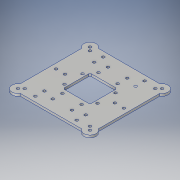
# Autodesk Inventor part: Piston Build frame
Saved by Autodesk Inventor 2018.1 (Build 221171000, 171)
## iProperties
Created: 2013-10-18
Part Number: Piston Build frame
Material: Aluminum 6061
Document SubType Name: Modeling
Designer: Gabriel Smolnycki
Mass: 160.206 g
Surface Area: 344.079 cm^2
Volume: 59.3356 cm^3
Density: 2.7 g/cm^3
Appearance: Aluminum - Flat
Sending System: SolidWorks 2017
Last Author: Gabriel Smolnycki
Last Saved: 2017-09-14
Author: Gabriel Smolnycki
Autodesk Inventor part; units mm, degrees
ref_plane "YZ Plane" through (0, 0, 0) normal (1, 0, 0) x (0, 1, 0)
ref_plane "XY Plane" through (0, 0, 0) normal (0, 0, 1) x (1, 0, 0)
ref_plane "Work Plane1" through (0, -4, 0) normal (0, 1, 0) x (-1, 0, 0)
sketch "Sketch1" plane through (0, -4, 0) normal (0, 1, 0) x (-1, 0, 0)
  arc A0 (65, 51.3397) -> (51.3397, 65) centre (60, 60) ccw
  line L0 (65, 51.3397) -> (65, -51.3397)
  arc A1 (51.3397, -65) -> (65, -51.3397) centre (60, -60) ccw
  line L1 (51.3397, -65) -> (-51.3397, -65)
  arc A2 (-65, -51.3397) -> (-51.3397, -65) centre (-60, -60) ccw
  line L2 (22.5, -20.5) -> (20.5, -22.5)
  line L3 (-65, -51.3397) -> (-65, 51.3397)
  arc A3 (-51.3397, 65) -> (-65, 51.3397) centre (-60, 60) ccw
  line L4 (22.5, 20.5) -> (22.5, -20.5)
  line L5 (20.5, 22.5) -> (22.5, 20.5)
  line L6 (-20.5, 22.5) -> (20.5, 22.5)
  line L7 (-22.5, 20.5) -> (-20.5, 22.5)
  line L8 (-51.3397, 65) -> (51.3397, 65)
  line L9 (-22.5, -20.5) -> (-22.5, 20.5)
  line L10 (-20.5, -22.5) -> (-22.5, -20.5)
  line L11 (20.5, -22.5) -> (-20.5, -22.5)
  constraints: 24 end point, 9 equal length, 8 point on circle, 4 centre point, 4 horizontal, 4 vertical, 3 equal radius, 1 perpendicular
extrude "Extrusion1" add sketch "Sketch1" along normal blind 4.064
hole "Hole32" at (34.5, 0.064, 56.5) direction (0, -1, 0) diameter 4.5 depth 4.064 tip angle 118
hole "Hole31" at (34.5, 0.064, 41.5) direction (0, -1, 0) diameter 4.5 depth 4.064 tip angle 118
hole "Hole30" at (56.5, 0.064, 0) direction (0, -1, 0) diameter 4.5 depth 4.064 tip angle 118
hole "Hole29" at (41.5, 0.064, 0) direction (0, -1, 0) diameter 4.5 depth 4.064 tip angle 118
hole "Hole28" at (34.5, 0, -41.5) direction (0, -1, 0) diameter 4.5 depth 4 tip angle 118
hole "Hole27" at (34.5, 0.064, -56.5) direction (0, -1, 0) diameter 4.5 depth 4.064 tip angle 118
hole "Hole26" at (-34.5, 0.064, -56.5) direction (0, -1, 0) diameter 4.5 depth 4.064 tip angle 118
hole "Hole25" at (-34.5, 0.064, -41.5) direction (0, -1, 0) diameter 4.5 depth 4.064 tip angle 118
hole "Hole24" at (-41.5, 0.064, 0) direction (0, -1, 0) diameter 4.5 depth 4.064 tip angle 118
hole "Hole23" at (-56.5, 0.064, 0) direction (0, -1, 0) diameter 4.5 depth 4.064 tip angle 118
hole "Hole22" at (-34.5, 0.064, 41.5) direction (0, -1, 0) diameter 4.5 depth 4.064 tip angle 118
hole "Hole21" at (-34.5, 0.064, 56.5) direction (0, -1, 0) diameter 4.5 depth 4.064 tip angle 118
hole "Hole20" at (-16, 0.064, -46) direction (0, -1, 0) diameter 4.5 depth 4.064 tip angle 118
hole "Hole19" at (-16, 0.064, -30) direction (0, -1, 0) diameter 4.5 depth 4.064 tip angle 118
hole "Hole18" at (16, 0.064, -30) direction (0, -1, 0) diameter 4.5 depth 4.064 tip angle 118
hole "Hole17" at (16, 0.064, -46) direction (0, -1, 0) diameter 4.5 depth 4.064 tip angle 118
sketch "Sketch17" plane through (0, 0.064, 0) normal (0, 1, 0) x (-1, 0, 0)
  point P0 (-16, -46)
hole "Hole16" at (16, 0.064, 46) direction (0, -1, 0) diameter 4.5 depth 4.064 tip angle 118
sketch "Sketch16" plane through (0, 0.064, 0) normal (0, 1, 0) x (-1, 0, 0)
  point P0 (-16, -30)
hole "Hole15" at (16, 0.064, 30) direction (0, -1, 0) diameter 4.5 depth 4.064 tip angle 118
sketch "Sketch15" plane through (0, 0.064, 0) normal (0, 1, 0) x (-1, 0, 0)
  point P0 (16, -30)
hole "Hole14" at (-16, 0.064, 30) direction (0, -1, 0) diameter 4.5 depth 4.064 tip angle 118
sketch "Sketch14" plane through (0, 0.064, 0) normal (0, 1, 0) x (-1, 0, 0)
  point P0 (16, -46)
hole "Hole13" at (-16, 0.064, 46) direction (0, -1, 0) diameter 4.5 depth 4.064 tip angle 118
sketch "Sketch13" plane through (0, 0.064, 0) normal (0, 1, 0) x (-1, 0, 0)
  point P0 (34.5, 56.5)
hole "Hole12" at (-27.5, 0.064, 15) direction (0, -1, 0) diameter 4.5 depth 4.064 tip angle 118
sketch "Sketch12" plane through (0, 0.064, 0) normal (0, 1, 0) x (-1, 0, 0)
  point P0 (34.5, 41.5)
hole "Hole11" at (-27.5, 0.064, -15) direction (0, -1, 0) diameter 4.5 depth 4.064 tip angle 118
sketch "Sketch11" plane through (0, 0.064, 0) normal (0, 1, 0) x (-1, 0, 0)
  point P0 (56.5, 0)
hole "Hole10" at (27.5, 0.064, -15) direction (0, -1, 0) diameter 4.5 depth 4.064 tip angle 118
sketch "Sketch10" plane through (0, 0.064, 0) normal (0, 1, 0) x (-1, 0, 0)
  point P0 (41.5, 0)
hole "Hole9" at (27.5, 0.064, 15) direction (0, -1, 0) diameter 4.5 depth 4.064 tip angle 118
sketch "Sketch9" plane through (0, 0.064, 0) normal (0, 1, 0) x (-1, 0, 0)
  point P0 (34.5, -41.5)
hole "Hole8" at (54.3431, 0.064, -54.3431) direction (0, -1, 0) diameter 4.5 depth 4.064 tip angle 118
sketch "Sketch8" plane through (0, 0.064, 0) normal (0, 1, 0) x (-1, 0, 0)
  point P0 (34.5, -56.5)
hole "Hole7" at (54.3431, 0.064, 54.3431) direction (0, -1, 0) diameter 4.5 depth 4.064 tip angle 118
sketch "Sketch7" plane through (0, 0.064, 0) normal (0, 1, 0) x (-1, 0, 0)
  point P0 (-34.5, -56.5)
hole "Hole6" at (-54.3431, 0.064, 54.3431) direction (0, -1, 0) diameter 4.5 depth 4.064 tip angle 118
sketch "Sketch6" plane through (0, 0, 0) normal (0, 1, 0) x (-1, 0, 0)
  point P0 (-34.5, -41.5)
hole "Hole5" at (-60, -4, 60) direction (0, 1, 0) diameter 4.5 depth 4.064 tip angle 118
sketch "Sketch5" plane through (0, 0.064, 0) normal (0, 1, 0) x (-1, 0, 0)
  point P0 (-41.5, 0)
hole "Hole4" at (60, -4, 60) direction (0, 1, 0) diameter 4.5 depth 4.064 tip angle 118
sketch "Sketch4" plane through (0, 0.064, 0) normal (0, 1, 0) x (-1, 0, 0)
  point P0 (-56.5, 0)
hole "Hole3" at (60, -4, -60) direction (0, 1, 0) diameter 4.5 depth 4.064 tip angle 118
sketch "Sketch3" plane through (0, 0.064, 0) normal (0, 1, 0) x (-1, 0, 0)
  point P0 (-34.5, 41.5)
hole "Hole2" at (-60, -4, -60) direction (0, 1, 0) diameter 4.5 depth 4.064 tip angle 118
sketch "Sketch2" plane through (0, 0.064, 0) normal (0, 1, 0) x (-1, 0, 0)
  point P0 (-34.5, 56.5)
hole "Hole1" at (-54.3431, 0.064, -54.3431) direction (0, -1, 0) diameter 4.5 depth 4.064 tip angle 118
sketch "Sketch18" plane through (0, 0.064, 0) normal (0, 1, 0) x (-1, 0, 0)
  point P0 (-16, 46)
sketch "Sketch19" plane through (0, 0.064, 0) normal (0, 1, 0) x (-1, 0, 0)
  point P0 (-16, 30)
sketch "Sketch20" plane through (0, 0.064, 0) normal (0, 1, 0) x (-1, 0, 0)
  point P0 (16, 30)
sketch "Sketch21" plane through (0, 0.064, 0) normal (0, 1, 0) x (-1, 0, 0)
  point P0 (16, 46)
sketch "Sketch22" plane through (0, 0.064, 0) normal (0, 1, 0) x (-1, 0, 0)
  point P0 (27.5, 15)
sketch "Sketch23" plane through (0, 0.064, 0) normal (0, 1, 0) x (-1, 0, 0)
  point P0 (27.5, -15)
sketch "Sketch24" plane through (0, 0.064, 0) normal (0, 1, 0) x (-1, 0, 0)
  point P0 (-27.5, -15)
sketch "Sketch25" plane through (0, 0.064, 0) normal (0, 1, 0) x (-1, 0, 0)
  point P0 (-27.5, 15)
sketch "Sketch26" plane through (0, 0.064, 0) normal (0, 1, 0) x (-1, 0, 0)
  point P0 (-54.3431, -54.3431)
sketch "Sketch27" plane through (0, 0.064, 0) normal (0, 1, 0) x (-1, 0, 0)
  point P0 (-54.3431, 54.3431)
sketch "Sketch28" plane through (0, 0.064, 0) normal (0, 1, 0) x (-1, 0, 0)
  point P0 (54.3431, 54.3431)
sketch "Sketch29" plane through (0, -4, 0) normal (0, 1, 0) x (-1, 0, 0)
  point P0 (60, 60)
sketch "Sketch30" plane through (0, -4, 0) normal (0, 1, 0) x (-1, 0, 0)
  point P0 (-60, 60)
sketch "Sketch31" plane through (0, -4, 0) normal (0, 1, 0) x (-1, 0, 0)
  point P0 (-60, -60)
sketch "Sketch32" plane through (0, -4, 0) normal (0, 1, 0) x (-1, 0, 0)
  point P0 (60, -60)
sketch "Sketch33" plane through (0, 0.064, 0) normal (0, 1, 0) x (-1, 0, 0)
  point P0 (54.3431, -54.3431)
body "Solid3"
